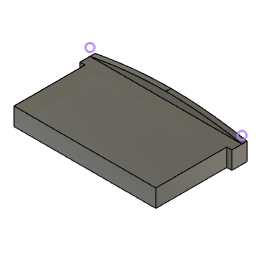
GBA_cassette_case top (Autodesk Fusion 360 archive; units mm, degrees)
design "GBA_cassette"
Autodesk Fusion 360 part; units mm, degrees
sketch "スケッチ1" plane through (0, 0, 0) normal (0, 0, 1) x (1, 0, 0)
  line L0 (0, 0) -> (60, 0)
  line L1 (60, 0) -> (60, 34)
  line L2 (60, 34) -> (0, 34)
  line L3 (0, 34) -> (0, 0)
  dimension "d1" = 60
  dimension "d2" = 34
  constraint horizontal L0
  constraint vertical L1
  constraint horizontal L2
  constraint vertical L3
  constraint coincident L0.start L3.end
  measures "d1" distance of L0.start L0.end
  measures "d2" distance of L0.start L2.end
extrude "押し出し1" add sketch "スケッチ1" along normal blind 10
sketch "スケッチ2" plane through (0, 0, 10) normal (0, 0, 1) x (-1, 0, 0)
  line L0 (0, -34) -> (0, 0)
  line L1 (0, 0) -> (-60, 0)
  line L2 (-60, 0) -> (-60, -34)
  line L3 (-60, -34) -> (0, -34)
  line L4 (-60, 0) -> (-58, 0)
  line L5 (-58, 0) -> (-58, -28)
  line L6 (-58, -28) -> (-60, -28)
  line L7 (-60, -28) -> (-60, 0)
  dimension "d5" = 2
  dimension "d6" = 28
  constraint horizontal L4
  constraint vertical L5
  constraint horizontal L6
  constraint vertical L7
  constraint coincident L1.end L2.start
  measures "d5" distance of L1.end L4.end
  measures "d6" distance of L1.end L6.end
extrude "押し出し2" cut sketch "スケッチ2" against normal blind 10 contours L1 L2 L4 L5 L6 L7
sketch "スケッチ3" plane through (0, 0, 10) normal (0, 0, 1) x (-1, 0, 0)
  line L0 (-58, 0) -> (-58, -28)
  line L1 (-58, -28) -> (-60, -28)
  line L2 (-60, -28) -> (-60, -34)
  line L3 (-60, -34) -> (0, -34)
  line L4 (0, -34) -> (0, 0)
  line L5 (0, 0) -> (-58, 0)
  line L6 (0, 0) -> (-2, 0)
  line L7 (-2, 0) -> (-2, -28)
  line L8 (-2, -28) -> (0, -28)
  line L9 (0, -28) -> (0, 0)
  dimension "d9" = 2
  dimension "d10" = 28
  constraint horizontal L6
  constraint vertical L7
  constraint horizontal L8
  constraint vertical L9
  constraint coincident L4.end L5.start
  measures "d9" distance of L4.end L6.end
  measures "d10" distance of L4.end L8.end
extrude "押し出し3" cut sketch "スケッチ3" against normal blind 15 contours L4 L5 L6 L7 L8 L9
sketch "スケッチ4" plane through (0, 0, 0) normal (0, 1, 0) x (1, 0, 0)
sketch "スケッチ5" plane through (0, 0, 0) normal (0, -1, 0) x (1, 0, 0)
  line L0 (2, 10) -> (2, 0)
  line L1 (2, 0) -> (58, 0)
  line L2 (58, 0) -> (58, 10)
  line L3 (58, 10) -> (2, 10)
  line L4 (58, 10) -> (2, 10)
  line L5 (2, 10) -> (2, 7)
  line L6 (2, 7) -> (58, 7)
  line L7 (58, 7) -> (58, 10)
  dimension "d13" = 3
  constraint horizontal L4
  constraint vertical L5
  constraint horizontal L6
  constraint vertical L7
  constraint coincident L2.end L3.start
  measures "d13" distance of L2.end L6.end
extrude "押し出し4" cut sketch "スケッチ5" against normal blind 32 contours L0 L2 L3 L4 L5 L6 L7
sketch "スケッチ6" plane through (0, 0, 10) normal (0, 0, 1) x (-1, 0, 0)
  line L0 (-2, -28) -> (-2, -32)
  line L1 (-2, -32) -> (-58, -32)
  line L2 (-58, -32) -> (-58, -28)
  line L3 (-58, -28) -> (-60, -28)
  line L4 (-60, -28) -> (-60, -34)
  line L5 (-60, -34) -> (0, -34)
  line L6 (0, -34) -> (0, -28)
  line L7 (0, -28) -> (-2, -28)
  line L8 (-2, -28) -> (0, -28)
  line L9 (0, -28) -> (0, -32)
  line L10 (0, -32) -> (-2, -32)
  line L11 (-2, -32) -> (-2, -28)
  constraint horizontal L8
  constraint vertical L9
  constraint horizontal L10
  constraint vertical L11
  constraint coincident L6 L9.end
  constraint coincident L0.start L7.end
extrude "押し出し5" cut sketch "スケッチ6" against normal blind 3 contours L0 L6 L7 L8 L9 L10 L11
sketch "スケッチ7" plane through (0, 0, 10) normal (0, 0, 1) x (-1, 0, 0)
  line L0 (0, -32) -> (-58, -32)
  line L1 (-58, -32) -> (-58, -28)
  line L2 (-58, -28) -> (-60, -28)
  line L3 (-60, -28) -> (-60, -34)
  line L4 (-60, -34) -> (0, -34)
  line L5 (0, -34) -> (0, -32)
  line L6 (-58, -32) -> (-60, -32)
  line L7 (-60, -32) -> (-60, -28)
  line L8 (-60, -28) -> (-58, -28)
  line L9 (-58, -28) -> (-58, -32)
  constraint horizontal L6
  constraint vertical L7
  constraint horizontal L8
  constraint vertical L9
  constraint coincident L2.end L3.start
  constraint coincident L0.end L1.start
extrude "押し出し6" cut sketch "スケッチ7" against normal blind 3 contours L1 L2 L3 L6 L7 L8 L9
sketch "スケッチ8" plane through (0, 0, 10) normal (0, 0, 1) x (-1, 0, 0)
  line L0 (-60, -32) -> (-60, -34)
  line L1 (-60, -34) -> (0, -34)
  line L2 (0, -34) -> (0, -32)
sketch "スケッチ9" plane through (0, 0, 10) normal (0, 0, 1) x (1, 0, 0)
sketch "スケッチ10" plane through (0, 32, 0) normal (0, -1, 0) x (1, 0, 0)
  line L0 (60, 10) -> (0, 10)
  line L1 (0, 10) -> (0, 7)
  line L2 (0, 7) -> (60, 7)
  line L3 (60, 7) -> (60, 10)
  spline S0 degree 5 poles (0, 7) (1.2, 7.2275) (3.6, 7.6628) (7.2, 8.256) (12, 8.9257) (18, 9.5472) (24, 9.9337) (30, 10.066) (36, 9.9337) (42, 9.5472) (48, 8.9257) (52.8, 8.256) (56.4, 7.6628) (58.8, 7.2275) (60, 7) knots 0 0 0 0 0 0 0.1 0.2 0.3 0.4 0.5 0.6 0.7 0.8 0.9 1 1 1 1 1 1
  point P0 (30, 10)
  constraint coincident L1.end L2.start
  constraint midpoint L0 P0
  constraint coincident L2.end L3.start
extrude "押し出し7" cut sketch "スケッチ10" against normal blind 16 contours L0 L3 S0 | L0 L1 S0
sketch "スケッチ11" plane through (0, 0, 0) normal (0, 0, -1) x (1, 0, 0)
  line L0 (2, -28) -> (0, -28)
  line L1 (0, -28) -> (0, -34)
  line L2 (0, -34) -> (60, -34)
  line L3 (60, -34) -> (60, -28)
  line L4 (60, -28) -> (58, -28)
  line L5 (58, -28) -> (58, 0)
  line L6 (58, 0) -> (2, 0)
  line L7 (2, 0) -> (2, -28)
